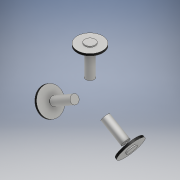
# Autodesk Inventor part: Motors and Wheels
Saved by Autodesk Inventor 2018 (Build 220112000, 112)
## iProperties
Created: 2018-09-04
Part Number: Motors and Wheels
Material: Generic
Document SubType Name: Modeling
Designer: matth
Density: 1 g/cm^3
Appearance: Default
Author: matth
Autodesk Inventor part; units mm, degrees
ref_plane "YZ Plane" through (0, 0, 0) normal (1, 0, 0) x (0, 1, 0)
ref_plane "XZ Plane" through (0, 0, 0) normal (0, 1, 0) x (-1, 0, 0)
ref_plane "XY Plane" through (0, 0, 0) normal (0, 0, 1) x (1, 0, 0)
sketch "Sketch1" plane through (0, 0, 0) normal (0, 1, 0) x (-1, 0, 0)
  line L0 (0, 0) -> (72.811086, -42.0375)
  line L1 (0, 0) -> (84.075, 0) construction
  line L2 (0, 0) -> (-72.811086, -42.0375)
  line L3 (0, 0) -> (84.075, 0) construction
  line L4 (0, 0) -> (0, 84.075)
  line L5 (72.811086, -42.0375) -> (77.141213, -44.5375)
  line L6 (77.141213, -44.5375) -> (75.641213, -47.135576)
  line L7 (75.641213, -47.135576) -> (71.311086, -44.635576)
  line L8 (71.311086, -44.635576) -> (72.811086, -42.0375)
  line L9 (-72.811086, -42.0375) -> (-77.141213, -44.5375)
  line L10 (-77.141213, -44.5375) -> (-78.641213, -41.939424)
  line L11 (-78.641213, -41.939424) -> (-74.311086, -39.439424)
  line L12 (-74.311086, -39.439424) -> (-72.811086, -42.0375)
  line L13 (0, 84.075) -> (0, 89.075)
  line L14 (0, 89.075) -> (-3, 89.075)
  line L15 (-3, 89.075) -> (-3, 84.075)
  line L16 (-3, 84.075) -> (0, 84.075)
  dimension "d0" = 84.075
  dimension "d1" = 30
  dimension "d2" = 84.075
  dimension "d3" = 150
  dimension "d4" = 84.075
  dimension "d5" = 5
  dimension "d6" = 3
  dimension "d7" = 3
  dimension "d8" = 5
  dimension "d9" = 3
  constraints: 34 end point, 6 parallel, 4 perpendicular, 2 equal length, 2 horizontal, 1 point on line, 1 vertical
  measures "d0" distance of L0.start L0.end
  measures "d1" angle of L0 L1
  measures "d2" distance of L0.start L2.end
  measures "d3" angle of L2 L3
  measures "d4" distance of L0.start L4.end
  measures "d5" distance of L0.end L5.end
  measures "d6" distance of L5.end L6.end
  measures "d7" distance of L9.end L10.end
  measures "d8" distance of L4.end L13.end
  measures "d9" distance of L14.end L13.end
revolve "Revolution1" add sketch "Sketch1" angle 360 about axis through (-72.811086, 0, -42.0375) along (-0.8660254, 0, -0.5) contours L5 L6 L7 L8
revolve "Revolution2" add sketch "Sketch1" angle 360 about axis through (0, 0, 84.075) along (0, 0, 1) contours L16 L15 L14 L13
revolve "Revolution3" add sketch "Sketch1" angle 360 about axis through (72.811086, 0, -42.0375) along (0.8660254, 0, -0.5) contours L9 L10 L11 L12
sketch "Sketch2" plane through (0, 0, 89.075) normal (0, 0, 1) x (1, 0, 0)
  circle A0 centre (0, 0) radius 3 projected
  circle A1 centre (0, 0) radius 25
  dimension "d13" = 50
  constraints: 1 centre point, 1 coincident
  measures "d13" diameter of A1
extrude "Extrusion1" add sketch "Sketch2" along normal blind 4
sketch "Sketch3" plane through (0, 0, 93.075) normal (0, 0, 1) x (1, 0, 0)
  circle A0 centre (0, 0) radius 10
  dimension "d16" = 20
  constraints: 1 centre point, 1 coincident
  measures "d16" diameter of A0
extrude "Extrusion2" add sketch "Sketch3" along normal blind 2
sketch "Sketch4" plane through (-77.141213, 0, -44.5375) normal (-0.8660254, 0, -0.5) x (-0.5, 0, 0.8660254)
  circle A0 centre (0, 0) radius 25
  dimension "d19" = 50
  constraints: 1 centre point, 1 coincident
  measures "d19" diameter of A0
extrude "Extrusion3" add sketch "Sketch4" along normal blind 4
sketch "Sketch5" plane through (-80.605314, 0, -46.5375) normal (-0.8660254, 0, -0.5) x (-0.5, 0, 0.8660254)
  circle A0 centre (0, 0) radius 10
  dimension "d22" = 20
  constraints: 1 centre point, 1 coincident
  measures "d22" diameter of A0
extrude "Extrusion4" add sketch "Sketch5" along normal blind 2
sketch "Sketch6" plane through (77.141213, 0, -44.5375) normal (0.8660254, 0, -0.5) x (-0.5, 0, -0.8660254)
  circle A0 centre (0, 0) radius 25
  dimension "d25" = 50
  constraints: 1 centre point, 1 coincident
  measures "d25" diameter of A0
extrude "Extrusion5" add sketch "Sketch6" along normal blind 4
sketch "Sketch7" plane through (80.605314, 0, -46.5375) normal (0.8660254, 0, -0.5) x (-0.5, 0, -0.8660254)
  circle A0 centre (0, 0) radius 10
  dimension "d28" = 20
  constraints: 1 centre point, 1 coincident
  measures "d28" diameter of A0
extrude "Extrusion6" add sketch "Sketch7" along normal blind 2
sketch "Sketch8" plane through (0, 0, 84.075) normal (0, 0, -1) x (-1, 0, 0)
  circle A0 centre (0, 0) radius 1.5
  dimension "d31" = 3
  constraints: 1 centre point, 1 coincident
  measures "d31" diameter of A0
extrude "Extrusion7" add sketch "Sketch8" along normal blind 3
sketch "Sketch9" plane through (0, 0, 81.075) normal (0, 0, -1) x (-1, 0, 0)
  circle A0 centre (0, 0) radius 8
  dimension "d34" = 16
  constraints: 1 centre point, 1 coincident
  measures "d34" diameter of A0
extrude "Extrusion8" add sketch "Sketch9" along normal blind 46
sketch "Sketch10" plane through (-72.811086, 0, -42.0375) normal (0.8660254, 0, 0.5) x (0.5, 0, -0.8660254)
  circle A0 centre (0, 0) radius 1.5
  dimension "d37" = 3
  constraints: 1 centre point, 1 coincident
  measures "d37" diameter of A0
extrude "Extrusion9" add sketch "Sketch10" along normal blind 3
sketch "Sketch11" plane through (-70.21301, 0, -40.5375) normal (0.8660254, 0, 0.5) x (0.5, 0, -0.8660254)
  circle A0 centre (0, 0) radius 8
  dimension "d40" = 16
  constraints: 1 centre point, 1 coincident
  measures "d40" diameter of A0
extrude "Extrusion10" add sketch "Sketch11" along normal blind 46
sketch "Sketch12" plane through (72.811086, 0, -42.0375) normal (-0.8660254, 0, 0.5) x (0.5, 0, 0.8660254)
  circle A0 centre (0, 0) radius 1.5
  dimension "d43" = 3
  constraints: 1 centre point, 1 coincident
  measures "d43" diameter of A0
extrude "Extrusion11" add sketch "Sketch12" along normal blind 3
sketch "Sketch13" plane through (70.21301, 0, -40.5375) normal (-0.8660254, 0, 0.5) x (0.5, 0, 0.8660254)
  circle A0 centre (0, 0) radius 8
  dimension "d46" = 16
  constraints: 1 centre point, 1 coincident
  measures "d46" diameter of A0
extrude "Extrusion12" add sketch "Sketch13" along normal blind 46
body "Solid1"
